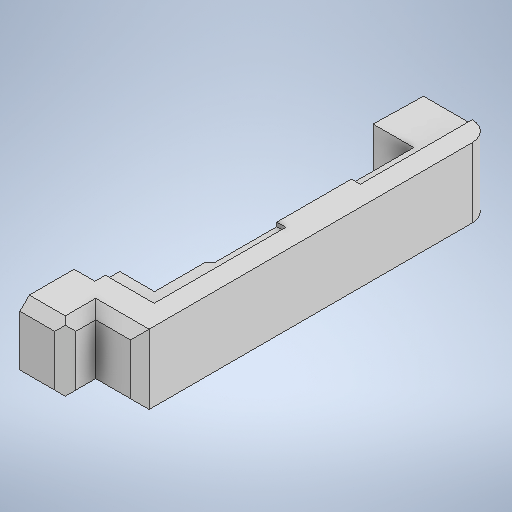
# Autodesk Inventor part: Part2
Saved by Autodesk Inventor 2025 (Build 290162000, 162)
## iProperties
Created: 2026-06-07
Part Number: Part2
Material: Generic
Document SubType Name: Modeling
Designer: user
Density: 1 g/cm^3
Appearance: Default
Author: user
Autodesk Inventor part; units mm, degrees
ref_plane "YZ Plane" through (0, 0, 0) normal (1, 0, 0) x (0, 1, 0)
ref_plane "XZ Plane" through (0, 0, 0) normal (0, 1, 0) x (-1, 0, 0)
ref_plane "XY Plane" through (0, 0, 0) normal (0, 0, 1) x (1, 0, 0)
sketch "Sketch1" plane through (0, 0, 0) normal (0, 1, 0) x (-1, 0, 0)
  line L0 (45, 192.5) -> (-45, 192.5)
  line L1 (-45, 192.5) -> (-45, -192.5)
  line L2 (-45, -192.5) -> (45, -192.5)
  line L3 (45, -192.5) -> (45, 192.5)
  line L4 (45, 192.5) -> (-45, -192.5) construction
  line L5 (-45, 192.5) -> (45, -192.5) construction
  line L6 (45, 138.0648) -> (24, 138.0648)
  line L7 (24, 138.0648) -> (24, 113.0648)
  line L8 (24, 113.0648) -> (-11, 113.0648)
  line L9 (-11, 113.0648) -> (-11, 62.0648)
  line L10 (-11, 62.0648) -> (-15.9497, 57.115)
  line L11 (-15.9497, 57.115) -> (-15.9497, -142.885)
  line L12 (-15.9497, -142.885) -> (25.0503, -142.885)
  line L13 (25.0503, -142.885) -> (24, -192.5)
  line L14 (-45, 151.0874) -> (10, 151.0874)
  line L15 (10, 151.0874) -> (10, 180.0874)
  line L16 (10, 180.0874) -> (45, 180.0874)
  line L17 (10, 192.5) -> (-0.6066, 181.8934)
  line L18 (-0.6066, 181.8934) -> (-0.6066, 161.8934)
  line L19 (-0.6066, 161.8934) -> (-35.6066, 161.8934)
  line L20 (-35.6066, 161.8934) -> (-46.4126, 151.0874)
  line L21 (-0.6066, 161.8934) -> (10, 151.0874)
  line L22 (10, 180.0874) -> (3.7937, 186.2937)
  point P0 (0, 0)
  point P1 (-45, 152.5)
  dimension "d0" = 90
  dimension "d1" = 385
  dimension "d25" = 21
  dimension "d27" = 25
  dimension "d28" = 35
  dimension "d29" = 51
  dimension "d30" = 7
  dimension "d31" = 135
  dimension "d32" = 200
  dimension "d33" = 41
  dimension "d34" = 55
  dimension "d35" = 29
  dimension "d36" = 15
  dimension "d37" = 20
  dimension "d38" = 35
  constraints: 46 end point, 10 perpendicular, 9 point on line, 6 parallel, 2 midpoint, 1 horizontal
  measures "d0" distance of L2.end L1.end
  measures "d1" distance of L1.end L0.end
  measures "d25" distance of L6.start L6.end
  measures "d27" distance of L6.end L7.end
  measures "d28" distance of L7.end L8.end
  measures "d29" distance of L8.end L9.end
  measures "d30" distance of L9.end L10.end
  measures "d31" angle of L9 L10
  measures "d32" distance of L10.end L11.end
  measures "d33" distance of L11.end L12.end
  measures "d34" distance of L14.start L14.end
  measures "d35" distance of L14.end L15.end
  measures "d36" distance of L17.start L17.end
  measures "d37" distance of L17.end L18.end
  measures "d38" distance of L18.end L19.end
extrude "Extrusion1" add sketch "Sketch1" along normal blind 70 contours L3 L16 L22 L17 L0 | L3 L6 L7 L8 L9 L10 L11 L12 L13 L2 L1 L14 L15 L16 | L22 L15 L21 L18 L17 | L20 L19 L21 L14 L1
fillet "Fillet1" radius 20 1 edges at (45, 35, -192.5)
sketch "Sketch2" plane through (0, 70, 0) normal (0, 1, 0) x (1, 0, 0)
  arc A0 (45, 172.5) -> (25, 192.5) centre (25, 172.5) ccw projected
  line L0 (45, 172.5) -> (25, 172.5)
  line L1 (25, 172.5) -> (25, -161.8934)
  line L2 (0.6066, -161.8934) -> (35.6066, -161.8934) projected
  line L3 (25, 172.5) -> (25, 192.5171)
  line L4 (25, 192.5171) -> (25, 80.0171)
  line L5 (25, 80.0171) -> (15.9497, 80.0171)
  line L6 (15.9497, 142.885) -> (15.9497, -57.115) projected
  line L7 (25, 80.0171) -> (25, 5.0171)
  line L8 (25, 5.0171) -> (15.9497, 5.0171)
  line L9 (15.9497, 80.0171) -> (15.9497, 5.0171)
  arc A1 (45, 172.5) -> (25, 192.5) centre (25, 172.5) ccw projected
  line L10 (25, 192.5) -> (-24, 192.5) projected
  line L11 (-24, 192.5) -> (-25.0503, 142.885) projected
  line L12 (-25.0503, 142.885) -> (15.9497, 142.885) projected
  line L13 (15.9497, 142.885) -> (15.9497, -57.115) projected
  line L14 (15.9497, -57.115) -> (11, -62.0648) projected
  line L15 (11, -62.0648) -> (11, -113.0648) projected
  line L16 (11, -113.0648) -> (-24, -113.0648) projected
  line L17 (-24, -113.0648) -> (-24, -138.0648) projected
  line L18 (-24, -138.0648) -> (-45, -138.0648) projected
  line L19 (-45, -138.0648) -> (-45, -192.5) projected
  line L20 (45, -152.5) -> (45, 172.5) projected
  line L21 (25, 5.0171) -> (25, -127.4829)
  line L22 (25, -127.4829) -> (-24, -127.4829)
  line L23 (-45, -192.5) -> (-10, -192.5) projected
  line L24 (-10, -192.5) -> (0.6066, -181.8934) projected
  line L25 (0.6066, -181.8934) -> (0.6066, -161.8934) projected
  line L26 (0.6066, -161.8934) -> (35.6066, -161.8934) projected
  line L27 (35.6066, -161.8934) -> (45, -152.5) projected
  point P0 (0, 0)
  dimension "d45" = 112.5
  dimension "d46" = 75
  dimension "d47" = 132.5
  constraints: 20 end point, 8 point on line, 4 perpendicular, 1 collinear, 1 horizontal
  measures "d45" distance of L3.end L4.end
  measures "d46" distance of L4.end L7.end
  measures "d47" distance of L7.end L21.end
extrude "Extrusion2" cut sketch "Sketch2" against normal blind 4 contours L3 L1 L5 L6 L12 L11 L10 | L1 L22 L17 L16 L15 L14 L6 L8
sketch "Sketch3" plane through (0, 0, 0) normal (0, -1, 0) x (1, 0, 0)
  line L0 (25, -192.5) -> (25, -80.0171) projected
  line L1 (25, -80.0171) -> (15.9497, -80.0171) projected
  line L2 (15.9497, -5.0171) -> (25, -5.0171) projected
  line L3 (25, -5.0171) -> (25, 127.4829) projected
  line L4 (25, 127.4829) -> (-24, 127.4829) projected
  arc A0 (25, -192.5) -> (45, -172.5) centre (25, -172.5) ccw projected
  line L5 (45, 152.5) -> (45, -172.5) projected
  line L6 (35.6066, 161.8934) -> (45, 152.5) projected
  line L7 (0.6066, 161.8934) -> (35.6066, 161.8934) projected
  line L8 (0.6066, 181.8934) -> (0.6066, 161.8934) projected
  line L9 (-10, 192.5) -> (0.6066, 181.8934) projected
  line L10 (-45, 192.5) -> (-10, 192.5) projected
  line L11 (-45, 138.0648) -> (-45, 192.5) projected
  line L12 (-24, 138.0648) -> (-45, 138.0648) projected
  line L13 (-24, 113.0648) -> (-24, 138.0648) projected
  line L14 (11, 113.0648) -> (-24, 113.0648) projected
  line L15 (11, 62.0648) -> (11, 113.0648) projected
  line L16 (15.9497, 57.115) -> (11, 62.0648) projected
  line L17 (15.9497, -142.885) -> (15.9497, 57.115) projected
  line L18 (-25.0503, -142.885) -> (15.9497, -142.885) projected
  line L19 (-24, -192.5) -> (-25.0503, -142.885) projected
  line L20 (25, -192.5) -> (-24, -192.5) projected
  point P0 (0, 0)
extrude "Extrusion3" cut sketch "Sketch3" against normal blind 4 contours L20 L19 L18 L17 L1 L0 | L17 L16 L15 L14 L13 L4 L3 L2
chamfer "Chamfer2" distance 9.3934 angle 45 1 edges at (18.1066, 70, 161.8934)
chamfer "Chamfer3" distance 9.3934 angle 45 2 edges at (0.6066, 70, 171.8934) (-27.5, 70, 192.5)
chamfer "Chamfer4" distance 9.3934 angle 45 1 edges at (18.1066, 0, 161.8934)
chamfer "Chamfer5" distance 9.3934 angle 45 2 edges at (0.6066, 0, 171.8934) (-27.5, 0, 192.5)
sketch "Sketch4" plane through (-45, 0, 138.0648) normal (-1, 0, 0) x (0, 0, 1)
  line L0 (0, 0) -> (0, 70) projected
  line L1 (0, 0) -> (54.4352, 70)
  line L2 (0, 70) -> (54.4352, 0)
  circle A0 centre (27.2176, 35) radius 18.5
  point P0 (-138.0648, 0)
  dimension "d64" = 37
  constraints: 4 end point, 1 centre point, 1 midpoint
  measures "d64" diameter of A0
extrude "Extrusion4" cut sketch "Sketch4" against normal blind 39 contours A0 L2 L1 | L1 L2 A0 | A0 L1 L2 | L1 A0 L2
body "Solid1"
